Autodesk Inventor part; units mm, degrees
(part 2 of 2)
sketch "Sketch4" plane through (110.769312, -25, 24.175211) normal (0.9848078, 0, -0.1736482) x (-0.1736482, 0, -0.9848078)
  circle A0 centre (10, 39) radius 1.5 projected
  circle A1 centre (10, 11) radius 1.5 projected
  point P0 (43.042824, 25)
extrude "Extrusion4" cut sketch "Sketch4" against normal through all
sketch "Sketch5" plane through (0, 0, 0) normal (0, 0, -1) x (-1, 0, 0)
  arc A0 (-105.234033, -12.72) -> (-97.582335, -41.396714) centre (0, 0) ccw
  arc A1 (-99.277389, -12) -> (-92.058806, -39.053504) centre (0, 0) ccw
  line L0 (-97.582335, -41.396714) -> (-92.058806, -39.053504)
  line L1 (-99.277389, -12) -> (-105.234033, -12.72)
  arc A2 (-92.058806, 39.053504) -> (-99.277389, 12) centre (0, 0) ccw
  arc A3 (-97.582335, 41.396714) -> (-105.234033, 12.72) centre (0, 0) ccw
  line L2 (-92.058806, 39.053504) -> (-97.582335, 41.396714)
  line L3 (-105.234033, 12.72) -> (-99.277389, 12)
  arc A4 (-97.47615, 41.134416) -> (-105.01129, 12.894532) centre (0, 0) ccw
  line L4 (-97.47615, 41.134416) -> (-92.320847, 38.947415)
  arc A5 (-92.320847, 38.947415) -> (-99.451746, 12.222531) centre (0, 0) ccw
  line L5 (-99.451746, 12.222531) -> (-105.01129, 12.894532)
  arc A6 (-105.01129, -12.894532) -> (-97.47615, -41.134416) centre (0, 0) ccw
  line L6 (-105.01129, -12.894532) -> (-99.451746, -12.222531)
  arc A7 (-99.451746, -12.222531) -> (-92.320847, -38.947415) centre (0, 0) ccw
  line L7 (-92.320847, -38.947415) -> (-97.47615, -41.134416)
  point P0 (0, 0)
  dimension "d21" = 0.2
  dimension "d22" = 0.2
  constraints: 8 end point, 8 point on circle, 4 centre point, 6 other
  measures "d21" radial gap between concentric circles of A3 A4
  measures "d22" radial gap between concentric circles of A0 A6
sketch "Sketch5 outline for Extrusion5" plane through (0, 0, 0) normal (0, 0, -1) x (-1, 0, 0)
  line L0 (-92.320847, 38.947415) -> (-97.47615, 41.134416)
  arc A0 (-99.451746, 12.222531) -> (-92.320847, 38.947415) centre (0, 0) cw
  line L1 (-105.01129, 12.894532) -> (-99.451746, 12.222531)
  arc A1 (-97.47615, 41.134416) -> (-105.01129, 12.894532) centre (0, 0) ccw
  line L2 (-99.451746, -12.222531) -> (-105.01129, -12.894532)
  arc A2 (-92.320847, -38.947415) -> (-99.451746, -12.222531) centre (0, 0) cw
  line L3 (-97.47615, -41.134416) -> (-92.320847, -38.947415)
  arc A3 (-105.01129, -12.894532) -> (-97.47615, -41.134416) centre (0, 0) ccw
extrude "Extrusion5" add sketch "Sketch5 outline for Extrusion5" along normal blind 4.5
body "Solid1"
